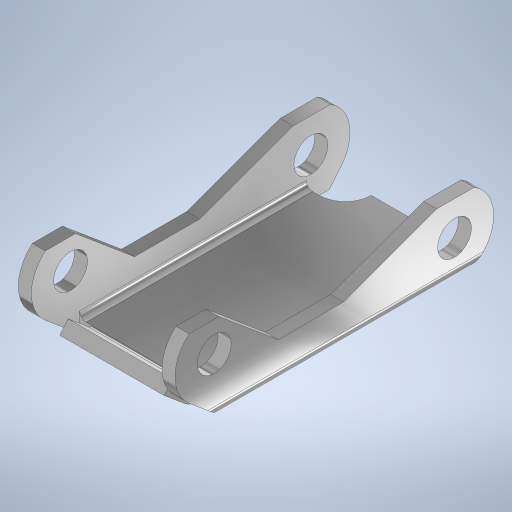
# Autodesk Inventor part: Lever
Saved by Autodesk Inventor 2024 (Build 280153000, 153)
## iProperties
Created: 2006-11-26
Document SubType Name: Modeling
Authority: Design by UAB Čeli APS
Material: Steel
Mass: 3.04941 g
Surface Area: 9.06896 cm^2
Volume: 0.388459 cm^3
Density: 7.85 g/cm^3
Appearance: Chrome - Polished
Pavadinimas: Aselė
Šifras: L-90.00 002
Mase: 0.00304941
Autodesk Inventor part; units mm, degrees
ref_plane "YZ Plane" through (0, 0, 0) normal (1, 0, 0) x (0, 1, 0)
ref_plane "XZ Plane" through (0, 0, 0) normal (0, 1, 0) x (-1, 0, 0)
ref_plane "XY Plane" through (0, 0, 0) normal (0, 0, 1) x (1, 0, 0)
sketch "Sketch2" plane through (0, 0, 0) normal (1, 0, 0) x (0, 1, 0)
  line L0 (0, 8.1606) -> (0, -1.3601) projected
  line L1 (-18.1996, 0) -> (16.4587, 0) construction
  arc A0 (-12.1735, 6.8) -> (-12.1757, 2.2019) centre (-10.2473, 4.5) ccw
  arc A1 (10.4508, 1.0716) -> (9.6493, 5.6) centre (8.1527, 3) ccw
  circle A2 centre (8.1527, 3) radius 1.3
  circle A3 centre (-10.2473, 4.5) radius 1.3
  line L2 (-0.3473, 3) -> (-5.3473, 3)
  line L3 (-9.5516, 0) -> (-12.1757, 2.2019)
  line L4 (9.5516, 0) -> (10.4508, 1.0716)
  line L5 (-9.5516, 0) -> (9.5516, 0)
  line L6 (-9.876, 6.8) -> (-5.3473, 3)
  line L7 (9.6493, 5.6) -> (6.7961, 5.6)
  line L8 (6.7961, 5.6) -> (-0.3473, 3)
  line L9 (-12.1735, 6.8) -> (-9.876, 6.8)
  point P0 (0, 0)
  dimension "d6" = 3
  dimension "d7" = 3
  dimension "d9" = 4.5
  dimension "d10" = 18.4
  dimension "d16" = 3
  dimension "d17" = 2.6
  dimension "d36" = 40
  dimension "d37" = 6.8
  dimension "d38" = 5.6
  dimension "d39" = 8.5
  dimension "d40" = 5
  dimension "d41" = 3
  dimension "d42" = 160
  dimension "d43" = 40
  constraints: 16 end point, 4 centre point, 4 point on circle, 3 point on line, 2 coincident, 2 parallel, 2 tangent, 1 equal radius, 1 midpoint, 1 perpendicular
  measures "d6" radius of A1
  measures "d7" distance from line of A1.centre L1
  measures "d9" distance from line of A0.centre L1
  measures "d10" horizontal distance of A0.centre A1.centre
  measures "d16" radius of A0
  measures "d17" diameter of A2
  measures "d36" angle of L1 L3
  measures "d37" distance between parallel lines of L9 L5
  measures "d38" distance between parallel lines of L7 L5
  measures "d39" distance of A2.centre L2.start
  measures "d40" distance of L2.start L2.end
  measures "d41" distance between parallel lines of L2 L5
  measures "d42" angle of L8 L2
  measures "d43" angle of L2 L6
extrude "Extrusion1" add sketch "Sketch2" along normal mid plane 12
shell "Shell1" thickness 1 removed faces 11 at (2, -12.3599, 2.37) at (2, 9.8602, 5.4667) at (2, 9.4358, 2.7915) at (2, -8.9642, 4.2915) at (2, -3.6807, 3) at (-2, -11.301, 1.4679) at (2, 10.1511, 0.7144) at (2, 2.0338, 3.8667) at (2, 7.7472, 5.6) at (-2, -6.8569, 4.2667) at (-2, -10.6418, 6.8)
fillet "Fillet2" radius 0.5 2 edges at (-5, -0.1763, 1) (5, -0.1763, 1)
fillet "Fillet3" radius 1 2 edges at (6, 0, 0) (-6, 0, 0)
sketch "Sketch5" plane through (6, -9.5516, 0) normal (0, 0, -1) x (-1, 0, 0)
  line L0 (1, 17.3423) -> (2, 17.3423)
  line L1 (10, 17.3423) -> (11, 17.3423)
  arc A0 (2, 17.3423) -> (4, 19.3423) centre (2, 19.3423) ccw
  arc A1 (8, 19.3423) -> (10, 17.3423) centre (10, 19.3423) ccw
  line L2 (4, 19.3423) -> (4, 20.5415)
  line L3 (4, 20.5415) -> (1, 20.5415)
  line L4 (8, 19.3423) -> (8, 20.5415)
  line L5 (8, 20.5415) -> (11, 20.5415)
  line L6 (1, 20.5415) -> (1, 17.3423)
  line L7 (11, 20.5415) -> (11, 17.3423)
  line L8 (1, -1.7876) -> (1, 20.3024) projected
  line L9 (11, 20.3024) -> (11, -1.7876) projected
  line L10 (10.5, 19.9423) -> (1.5, 19.9423) projected
  point P0 (6, -9.8516)
  dimension "d47" = 2
  dimension "d53" = 3.1991
  dimension "d54" = 3
  dimension "d55" = 3.1991
  dimension "d56" = 3
  dimension "d57" = 2
  dimension "d58" = 2.6
  constraints: 16 end point, 4 perpendicular, 4 point on circle, 4 tangent, 3 collinear, 2 centre point, 1 equal radius, 1 parallel
  measures "d47" radius of A0
  measures "d53" distance between parallel lines of L0 L3
  measures "d54" distance between parallel lines of L2 L6
  measures "d55" distance between parallel lines of L1 L5
  measures "d56" distance between parallel lines of L4 L7
  measures "d57" radius of A1
  measures "d58" distance between parallel lines of L0 L10
extrude "Extrusion4" cut sketch "Sketch5" against normal up to next
sketch "Sketch7" plane through (-4.5, -10.7434, 1) normal (0, 0, 1) x (1, 0, 0)
  line L0 (6.5, 20.5341) -> (6.5, 21.1341) projected
  line L1 (2.5, 21.1341) -> (6.5, 21.1341) projected
  line L2 (-0.5, 1.1918) -> (11.5, 1.1918) projected
  line L3 (6.5, 20.295) -> (2.5, 20.295) projected
  line L4 (-0.5, 1.1918) -> (9.5, 1.1918)
  line L5 (9.5, 1.1918) -> (9.5, -0.8082)
  line L6 (9.5, -0.8082) -> (-0.5, -0.8082)
  line L7 (-0.5, -0.8082) -> (-0.5, 1.1918)
  line L8 (-0.5, -1.4301) -> (-0.5, 0.8674) projected
  line L9 (2.5, 21.1341) -> (6.5, 21.1341)
  line L10 (6.5, 21.1341) -> (6.5, 20.5341)
  line L11 (6.5, 20.5341) -> (2.5, 20.5341)
  line L12 (2.5, 20.5341) -> (2.5, 21.1341)
  point P0 (2.5, 20.5341)
  point P1 (4.5, 10.7434)
  point P2 (9.5, -0.5959)
  dimension "d52" = 2
  constraints: 16 end point, 4 parallel, 3 point on line, 2 horizontal, 2 perpendicular, 1 horizontal alignment
  measures "d52" distance between parallel lines of L6 L2
extrude "Extrusion5" cut sketch "Sketch7" along normal through all both and the other way through all
sketch "Sketch8" plane through (0, 0, 0) normal (1, 0, 0) x (0, 1, 0)
  line L0 (-9.5516, 1) -> (7.7907, 1) projected
  line L1 (-9.5516, 0) -> (9.5516, 0) projected
  line L2 (-12.0753, 1.6595) -> (-11.4325, 2.4256)
  line L3 (-9.5516, 1) -> (-9.5516, 0)
  line L4 (-11.4325, 2.4256) -> (-9.873, 1.117)
  arc A0 (-9.873, 1.117) -> (-9.5516, 1) centre (-9.5516, 1.5) ccw
  line L5 (-12.0753, 1.6595) -> (-10.5158, 0.3509)
  arc A1 (-10.5158, 0.3509) -> (-9.5516, 0) centre (-9.5516, 1.5) ccw
  point P0 (0, 0)
  dimension "d61" = 50
  dimension "d62" = 1
  dimension "d63" = 1.5
  dimension "d64" = 3
  constraints: 8 end point, 4 point on circle, 4 tangent, 2 centre point, 2 perpendicular, 1 parallel
  measures "d61" angle of L4 L3
  measures "d62" distance between parallel lines of L5 L4
  measures "d63" distance from line of A0.centre L1
  measures "d64" distance from line of L1.start L2
extrude "Extrusion6" add sketch "Sketch8" along normal mid plane 8
body "Solid1"
